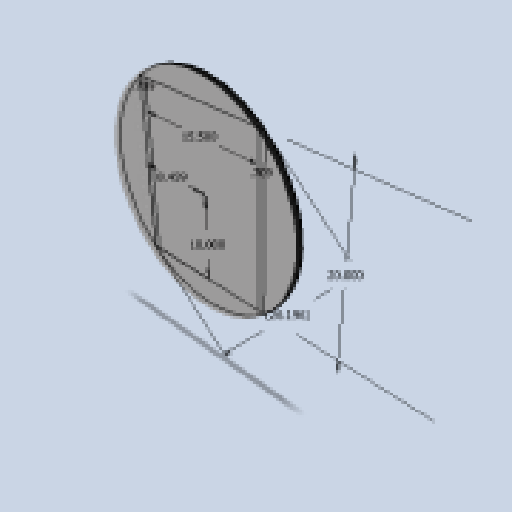
# Autodesk Inventor part: base turntable
Saved by Autodesk Inventor 2023 (Build 270158000, 158)
## iProperties
Created: 2022-10-13
Part Number: base turntable
Material: Generic
Document SubType Name: Modeling
Designer: Nathan
Density: 1 g/cm^3
Appearance: Default
Author: Nathan
Autodesk Inventor part; units mm, degrees
ref_plane "YZ Plane" through (0, 0, 0) normal (1, 0, 0) x (0, 1, 0)
ref_plane "XZ Plane" through (0, 0, 0) normal (0, 1, 0) x (-1, 0, 0)
ref_plane "XY Plane" through (0, 0, 0) normal (0, 0, 1) x (1, 0, 0)
sketch "Sketch1" plane through (0, 0, 0) normal (0, 0, 1) x (1, 0, 0)
  line L0 (0, 0) -> (429.7172, 0)
  line L1 (429.7172, 0) -> (429.7172, 508)
  line L2 (429.7172, 508) -> (0, 508)
  line L3 (0, 508) -> (0, 0)
  line L4 (18.0086, 508) -> (18.0086, 0)
  line L5 (411.7086, 508) -> (411.7086, 0)
  circle A0 centre (214.8586, 254) radius 332.6864
  point P0 (0, 254)
  dimension "d1" = 508
  dimension "d3" = 18.0086
  dimension "d4" = 18.0086
  dimension "d6" = 393.7
  dimension "d10" = 665.3727
  dimension "d13" = 214.8586
  dimension "d14" = 254
  constraints: 12 end point, 4 point on line, 3 parallel, 2 perpendicular, 1 horizontal, 1 midpoint, 3 other
  measures "d1" distance of L1.end L0.end
  measures "d3" distance between parallel lines of L3 L4
  measures "d4" distance between parallel lines of L1 L5
  measures "d6" distance between parallel lines of L5 L4
  measures "d10" distance of L0.start L1.end
  measures "d13" horizontal distance of L0.start point (214.859, 254)
  measures "d14" vertical distance of L0.start point (214.859, 254)
extrude "Extrusion2" add sketch "Sketch1" along normal blind 18.0086 contours A0 L3 | L0 A0 | L4 L2 L5 L0 | A0 L2 | L1 A0
extrude "Extrusion3" add sketch "Sketch1" along normal blind 17.78 contours L3 L2 L4 L0 | L0 L5 L2 L1
body "Solid2"
